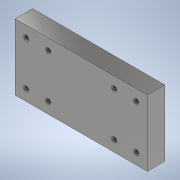
# Autodesk Inventor part: suporte topo
Saved by Autodesk Inventor 2021 (Build 250183000, 183)
## iProperties
Created: 2023-11-09
Part Number: suporte topo
Material: Genérico
Document SubType Name: Modeling
Designer: Vinic
Density: 1 g/cm^3
Appearance: Usinado 02
Author: Vinic
Autodesk Inventor part; units mm, degrees
ref_plane "YZ Plane" through (0, 0, 0) normal (1, 0, 0) x (0, 1, 0)
ref_plane "XZ Plane" through (0, 0, 0) normal (0, 1, 0) x (-1, 0, 0)
ref_plane "XY Plane" through (0, 0, 0) normal (0, 0, 1) x (1, 0, 0)
sketch "Esboço1" plane through (0, 0, 0) normal (0, 0, 1) x (1, 0, 0)
  line L0 (-300, -150) -> (300, -150)
  line L1 (300, -150) -> (300, 150)
  line L2 (300, 150) -> (-300, 150)
  line L3 (-300, 150) -> (-300, -150)
  line L4 (-300, -150) -> (300, 150) construction
  line L5 (300, -150) -> (-300, 150) construction
  point P0 (0, 0)
  dimension "d0" = 600
  dimension "d1" = 300
  constraints: 12 end point, 2 midpoint, 2 parallel, 1 horizontal, 1 perpendicular
  measures "d0" distance of L0.start L0.end
  measures "d1" distance of L0.end L1.end
extrude "Extrusão1" add sketch "Esboço1" along normal blind 80
sketch "Esboço2" plane through (0, 0, 80) normal (0, 0, 1) x (1, 0, 0)
  line L0 (-250, -100) -> (250, -100)
  line L1 (250, -100) -> (250, 100)
  line L2 (250, 100) -> (-250, 100)
  line L3 (-250, 100) -> (-250, -100)
  line L4 (-250, -100) -> (250, 100) construction
  line L5 (250, -100) -> (-250, 100) construction
  line L6 (-150, -100) -> (150, -100)
  line L7 (150, -100) -> (150, 100)
  line L8 (150, 100) -> (-150, 100)
  line L9 (-150, 100) -> (-150, -100)
  line L10 (-150, -100) -> (150, 100) construction
  line L11 (150, -100) -> (-150, 100) construction
  circle A0 centre (-250, 100) radius 8
  circle A1 centre (-150, 100) radius 8
  circle A2 centre (150, 100) radius 8
  circle A3 centre (250, 100) radius 8
  circle A4 centre (250, -100) radius 8
  circle A5 centre (150, -100) radius 8
  circle A6 centre (-150, -100) radius 8
  circle A7 centre (-250, -100) radius 8
  point P0 (0, 0)
  dimension "d4" = 500
  dimension "d5" = 200
  dimension "d6" = 300
  dimension "d7" = 16
  dimension "d8" = 16
  dimension "d9" = 16
  dimension "d10" = 16
  dimension "d11" = 16
  dimension "d12" = 16
  dimension "d13" = 16
  dimension "d14" = 16
  constraints: 24 end point, 8 centre point, 8 coincident, 4 midpoint, 4 parallel, 2 horizontal, 2 perpendicular, 1 point on line
  measures "d4" distance of L2.end L1.end
  measures "d5" distance of L2.end L0.start
  measures "d6" distance of L8.end L7.end
  measures "d7" diameter of A0
  measures "d8" diameter of A1
  measures "d9" diameter of A2
  measures "d10" diameter of A3
  measures "d11" diameter of A4
  measures "d12" diameter of A5
  measures "d13" diameter of A6
  measures "d14" diameter of A7
extrude "Extrusão2" cut sketch "Esboço2" against normal blind 40 contours L3 A7 L0 | L0 A7 L3 | A6 L9 L0 | L0 A6 | A0 L2 L3 | L3 L2 A0 | L9 A6 L0 | A1 L2 L9 | L9 L2 A1 | A5 L7 L0 | L0 A5 | A1 L2 | L7 A5 L0 | A2 L2 | L2 L7 A2 | L7 L2 A2 | A4 L1 L0 | L0 L1 A4 | A3 L1 L2 | L2 L1 A3
chamfer "Chanfro1" distance 4 angle 45 8 edges at (-258, 100, 80) (-158, 100, 80) (-258, -100, 80) (-158, -100, 80) (142, 100, 80) (142, -100, 80) (242, 100, 80) (242, -100, 80)
